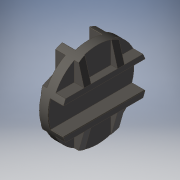
# Autodesk Inventor part: 60199320_1_20_20
Saved by Autodesk Inventor 2019 (Build 230136000, 136)
## iProperties
Created: 2024-03-16
Part Number: 60199320_1_20_20
Material: Generic
Catalog Web Link: www.cadenas.de
Description: kreuzsch_kpl_hzd_rf-Sliding disc, Torsionally-Stiff Couplings HZD with Through Holes, Stainless, Set-Srew Style
Vendor: MAEDLER
Document SubType Name: Modeling
Designer: psAdmin
Manufacturer: MAEDLER
Mass: 14.1613 g
Surface Area: 76.9254 cm^2
Volume: 14.1613 cm^3
Density: 1 g/cm^3
Appearance: PSOLRGB-222-219-214
Category: PARTsolutions
Company: MAEDLER
Title: 60199320
Author: Cadenas PARTsolutions
Comments: Sliding disc, Torsionally-Stiff Couplings HZD with Through Holes, Stainless, Set-Srew Style
PSOL_IDENT_0: {$CADENAS_DATA/23d-libs/maedler/antriebselemente/kupplungen/drehstarre_kupplungen/dr_k_hzd_m_db_rf/k
PSOL_IDENT_1: reuzsch_kpl_hzd_rf.prj},192 {VTYP=3D},{NB=60199320_1_20_20},{LINA=60199320},{NN=kreuzsch_kpl_hzd_rf}
PSOL_IDENT_2: ,{DATE=09.12.2023 00:25:54},{GEOMDATE=01.12.2023 07:25:45},{VERSION=},{LINEID=230},{WBVAR=BX1,BX2},{
PSOL_IDENT_3: WBNUMERIC=BX1,BX2}  {NB=60199320_1_20_20},{LINA=60199320},{KT=DUMMY},{ARTNR=60199320},{WEBSHOP=Produ
PSOL_IDENT_4: ktdetails / Katalogseite / Montageanleitung},{MATK=Edelstahl},{MAT=Naben aus Edelstahl rostfrei 1.43
PSOL_IDENT_5: 05 (V2A), Übertragungselement (Kreuzscheibe) aus schwarzem Polyacetal},{DM=30},{SBM=95},{B=20},{BMAX=
PSOL_IDENT_6: 25},{BX1=20.000},{BX2=20.000},{L1=59.6},{L2=20.6},{L3=18.4},{D1=50.0},{MVW=±0.5},{MVR=±0.25},{VS=137
PSOL_IDENT_7: 5},{GEW=510},{ARTNR1=60125000},{GEW1=20.0},{L4=20.6},{L5=29.00},{B1=15.4},{AB=42.65},{G=8},{AZ=2},{K
PSOL_IDENT_8: B=16.6},{KB2=23.4},{KB3=22.0},{KB4=15.45},{KTF=7.50},{KFT2=5.750},{KFT3=3.85},{KFT4=3.85},{TN=kreuzs
PSOL_IDENT_9: ch_kpl_hzd_rf_50.0_20},{CTN=84836080},{DIST=2.883333}
NB: 60199320_1_20_20
NN: kreuzsch_kpl_hzd_rf
NT: Sliding disc, Torsionally-Stiff Couplings HZD with Through Holes, Stainless, Set-Srew Style
NBSYN: $ARTNR._1_$BX1._$BX2.
LINA: 60199320
CATALOG: Mädler
ARTNR: 60199320
WEBSHOP: Product details / Catalogue page / Assembly instructions
MATK: Edelstahl
MAT: Hubs made from stainless steel 1.4305 (AISI 303), Torque disc made from black polyacetal
DM: 30
SBM: 95
B: 20
BMAX: 25
BX1: 20
BX2: 20
L1: 59.6
L2: 20.6
L3: 18.4
D1: 50
MVW: ±0.5
MVR: ±0.25
VS: 1375
GEW: 510
ARTNR1: 60125000
GEW1: 20
L4: 20.6
L5: 29
B1: 15.4
AB: 42.65
G: 8
AZ: 2
KB: 16.6
KB2: 23.4
KB3: 22
KB4: 15.45
KTF: 7.5
KFT2: 5.75
KFT3: 3.85
KFT4: 3.85
TN: kreuzsch_kpl_hzd_rf_50.0_20
CTN: 84836080
SUPPLIER: MAEDLER
ARTICLENO: 60199320_1_20_20
BOMINFO: 60199320
CREATOR: CADENAS GmbH
Autodesk Inventor part; units mm, degrees
ref_plane "YZ Plane" through (0, 0, 0) normal (1, 0, 0) x (0, 1, 0)
ref_plane "XZ Plane" through (0, 0, 0) normal (0, 1, 0) x (-1, 0, 0)
ref_plane "XY Plane" through (0, 0, 0) normal (0, 0, 1) x (1, 0, 0)
sketch "Sketch_3" plane through (0, 0, 0) normal (0, 0, 1) x (1, 0, 0)
  line L0 (8.3, 0) -> (-8.3, 0)
  line L1 (-8.3, 0) -> (-8.3, 25)
  line L2 (-8.3, 25) -> (8.3, 25)
  line L3 (8.3, 25) -> (8.3, 0)
  line L4 (8.3, 0) -> (-8.3, 0)
  constraints: 10 end point
revolve "Revolution1" add sketch "Sketch_3" angle 360 about axis through (8.3, 0, 0) along (1, 0, 0)
sketch "Sketch_4" plane through (-8.3, 0, 0) normal (1, 0, 0) x (0, 0, -1)
  line L0 (-7.7, 23.784659) -> (-7.7, -23.784659)
  arc A0 (-7.7, -23.784659) -> (7.7, -23.784659) centre (0, 0) ccw
  line L1 (7.7, -23.784659) -> (7.7, 23.784659)
  arc A1 (7.7, 23.784659) -> (-7.7, 23.784659) centre (0, 0) ccw
  constraints: 4 end point, 4 point on circle, 2 centre point
extrude "Extrusion1" cut sketch "Sketch_4" along normal blind 7.5
sketch "Sketch_12" plane through (-8.3, 0, 0) normal (1, 0, 0) x (0, 0, -1)
  line L0 (11.7, 22.093212) -> (11.7, 11)
  line L1 (11.7, 11) -> (22.449944, 11)
  arc A0 (22.449944, 11) -> (11.7, 22.093212) centre (0, 0) ccw
  constraints: 4 end point, 2 point on circle, 1 centre point
extrude "Extrusion2" cut sketch "Sketch_12" along normal blind 5.75
sketch "Sketch_13" plane through (-8.3, 0, 0) normal (1, 0, 0) x (0, 0, -1)
  line L0 (-22.449944, 11) -> (-11.7, 11)
  line L1 (-11.7, 11) -> (-11.7, 22.093212)
  arc A0 (-11.7, 22.093212) -> (-22.449944, 11) centre (0, 0) ccw
  constraints: 4 end point, 2 point on circle, 1 centre point
extrude "Extrusion3" cut sketch "Sketch_13" along normal blind 5.75
sketch "Sketch_14" plane through (-8.3, 0, 0) normal (1, 0, 0) x (0, 0, -1)
  arc A0 (11.7, -22.093212) -> (22.449944, -11) centre (0, 0) ccw
  line L0 (22.449944, -11) -> (11.7, -11)
  line L1 (11.7, -11) -> (11.7, -22.093212)
  constraints: 4 end point, 2 point on circle, 1 centre point
extrude "Extrusion4" cut sketch "Sketch_14" along normal blind 5.75
sketch "Sketch_15" plane through (-8.3, 0, 0) normal (1, 0, 0) x (0, 0, -1)
  arc A0 (-22.449944, -11) -> (-11.7, -22.093212) centre (0, 0) ccw
  line L0 (-11.7, -22.093212) -> (-11.7, -11)
  line L1 (-11.7, -11) -> (-22.449944, -11)
  constraints: 4 end point, 2 point on circle, 1 centre point
extrude "Extrusion5" cut sketch "Sketch_15" along normal blind 5.75
sketch "Sketch_16" plane through (-8.3, 0, 0) normal (1, 0, 0) x (0, 0, -1)
  line L0 (11.7, 7.725) -> (11.7, -7.725)
  line L1 (11.7, -7.725) -> (23.776551, -7.725)
  arc A0 (23.776551, -7.725) -> (23.776551, 7.725) centre (0, 0) ccw
  line L2 (23.776551, 7.725) -> (11.7, 7.725)
  constraints: 6 end point, 2 point on circle, 1 centre point
extrude "Extrusion6" cut sketch "Sketch_16" along normal blind 3.85
sketch "Sketch_17" plane through (-8.3, 0, 0) normal (1, 0, 0) x (0, 0, -1)
  arc A0 (-23.776551, 7.725) -> (-23.776551, -7.725) centre (0, 0) ccw
  line L0 (-23.776551, -7.725) -> (-11.7, -7.725)
  line L1 (-11.7, -7.725) -> (-11.7, 7.725)
  line L2 (-11.7, 7.725) -> (-23.776551, 7.725)
  constraints: 6 end point, 2 point on circle, 1 centre point
extrude "Extrusion7" cut sketch "Sketch_17" along normal blind 3.85
sketch "Sketch_18" plane through (8.3, 0, 0) normal (1, 0, 0) x (0, 0, -1)
  arc A0 (-23.784659, 7.7) -> (-23.784659, -7.7) centre (0, 0) ccw
  line L0 (-23.784659, -7.7) -> (23.784659, -7.7)
  arc A1 (23.784659, -7.7) -> (23.784659, 7.7) centre (0, 0) ccw
  line L1 (23.784659, 7.7) -> (-23.784659, 7.7)
  constraints: 4 end point, 4 point on circle, 2 centre point
extrude "Extrusion8" cut sketch "Sketch_18" against normal blind 7.5
sketch "Sketch_19" plane through (8.3, 0, 0) normal (1, 0, 0) x (0, 0, -1)
  line L0 (11.7, 22.093212) -> (11.7, 11)
  line L1 (11.7, 11) -> (22.449944, 11)
  arc A0 (22.449944, 11) -> (11.7, 22.093212) centre (0, 0) ccw
  constraints: 4 end point, 2 point on circle, 1 centre point
extrude "Extrusion9" cut sketch "Sketch_19" against normal blind 5.75
sketch "Sketch_20" plane through (8.3, 0, 0) normal (1, 0, 0) x (0, 0, -1)
  line L0 (-22.449944, 11) -> (-11.7, 11)
  line L1 (-11.7, 11) -> (-11.7, 22.093212)
  arc A0 (-11.7, 22.093212) -> (-22.449944, 11) centre (0, 0) ccw
  constraints: 4 end point, 2 point on circle, 1 centre point
extrude "Extrusion10" cut sketch "Sketch_20" against normal blind 5.75
sketch "Sketch_21" plane through (8.3, 0, 0) normal (1, 0, 0) x (0, 0, -1)
  arc A0 (11.7, -22.093212) -> (22.449944, -11) centre (0, 0) ccw
  line L0 (22.449944, -11) -> (11.7, -11)
  line L1 (11.7, -11) -> (11.7, -22.093212)
  constraints: 4 end point, 2 point on circle, 1 centre point
extrude "Extrusion11" cut sketch "Sketch_21" against normal blind 5.75
sketch "Sketch_22" plane through (8.3, 0, 0) normal (1, 0, 0) x (0, 0, -1)
  arc A0 (-22.449944, -11) -> (-11.7, -22.093212) centre (0, 0) ccw
  line L0 (-11.7, -22.093212) -> (-11.7, -11)
  line L1 (-11.7, -11) -> (-22.449944, -11)
  constraints: 4 end point, 2 point on circle, 1 centre point
extrude "Extrusion12" cut sketch "Sketch_22" against normal blind 5.75
sketch "Sketch_23" plane through (8.3, 0, 0) normal (1, 0, 0) x (0, 0, -1)
  line L0 (-7.725, 23.776551) -> (-7.725, 11)
  line L1 (-7.725, 11) -> (7.725, 11)
  line L2 (7.725, 11) -> (7.725, 23.776551)
  arc A0 (7.725, 23.776551) -> (-7.725, 23.776551) centre (0, 0) ccw
  constraints: 6 end point, 2 point on circle, 1 centre point
extrude "Extrusion13" cut sketch "Sketch_23" against normal blind 3.85
sketch "Sketch_24" plane through (8.3, 0, 0) normal (1, 0, 0) x (0, 0, -1)
  arc A0 (-7.725, -23.776551) -> (7.725, -23.776551) centre (0, 0) ccw
  line L0 (7.725, -23.776551) -> (7.725, -11)
  line L1 (7.725, -11) -> (-7.725, -11)
  line L2 (-7.725, -11) -> (-7.725, -23.776551)
  constraints: 6 end point, 2 point on circle, 1 centre point
extrude "Extrusion14" cut sketch "Sketch_24" against normal blind 3.85
sketch "Sketch_25" plane through (0, 0, 0) normal (0, 0, 1) x (1, 0, 0)
  line L0 (4.45, 25) -> (4.45, 24.600762)
  line L1 (4.45, 24.600762) -> (8.3, 11)
  line L2 (8.3, 11) -> (8.3, 25)
  line L3 (8.3, 25) -> (4.45, 25)
  constraints: 8 end point
extrude "Extrusion15" cut sketch "Sketch_25" along normal mid plane 23.4
sketch "Sketch_26" plane through (0, 0, 0) normal (0, 0, 1) x (1, 0, 0)
  line L0 (4.45, -25) -> (8.3, -25)
  line L1 (8.3, -25) -> (8.3, -11)
  line L2 (8.3, -11) -> (4.45, -24.600762)
  line L3 (4.45, -24.600762) -> (4.45, -25)
  constraints: 8 end point
extrude "Extrusion16" cut sketch "Sketch_26" along normal mid plane 23.4
sketch "Sketch_27" plane through (0, 0, 0) normal (0, 1, 0) x (1, 0, 0)
  line L0 (-8.3, 25) -> (-8.3, 11.7)
  line L1 (-8.3, 11.7) -> (-4.45, 24.600762)
  line L2 (-4.45, 24.600762) -> (-4.45, 25)
  line L3 (-4.45, 25) -> (-8.3, 25)
  constraints: 8 end point
extrude "Extrusion17" cut sketch "Sketch_27" along normal mid plane 22
sketch "Sketch_28" plane through (0, 0, 0) normal (0, 1, 0) x (1, 0, 0)
  line L0 (-8.3, -25) -> (-4.45, -25)
  line L1 (-4.45, -25) -> (-4.45, -24.600762)
  line L2 (-4.45, -24.600762) -> (-8.3, -11.7)
  line L3 (-8.3, -11.7) -> (-8.3, -25)
  constraints: 8 end point
extrude "Extrusion18" cut sketch "Sketch_28" along normal mid plane 22
chamfer "Chamfer1" distance 0.25 angle 45 8 edges at (4.55, 7.7, 23.7847) (4.55, 7.7, -23.7847) (0.8, 0, 25) (0.8, 0, -25) (4.55, -7.7, 23.7847) (4.55, -7.7, -23.7847) (8.3, 7.7, 0) (8.3, -7.7, 0)
chamfer "Chamfer2" distance 0.25 angle 45 9 edges at (-0.8, 24.6943, -3.8977) (-0.8, 24.6943, 3.8977) (-0.8, -25, 0) (-4.55, -23.7847, -7.7) (-4.55, 23.7847, -7.7) (-8.3, 0, -7.7) (-4.55, 23.7847, 7.7) (-4.55, -23.7847, 7.7) (-8.3, 0, 7.7)
ref_plane "center_1_XY" through (0, 0, 0) normal (1, 0, 0) x (0, 0, -1)
ref_plane "center_1_YZ" through (0, 0, 0) normal (0, 0, -1) x (0, 1, 0)
ref_plane "center_1_ZX" through (0, 0, 0) normal (0, 1, 0) x (1, 0, 0)
ref_plane "center_2_XY" through (0, 0, 0) normal (1, 0, 0) x (0, 0, -1)
ref_plane "center_2_YZ" through (0, 0, 0) normal (0, 0, -1) x (0, 1, 0)
ref_plane "center_2_ZX" through (0, 0, 0) normal (0, 1, 0) x (1, 0, 0)
body "Solid1"
